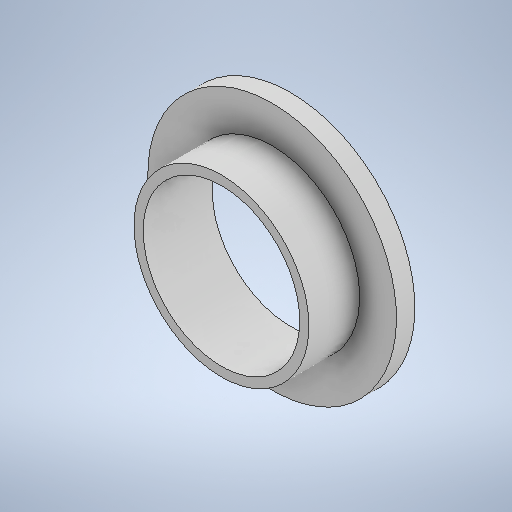
# Autodesk Inventor part: Ø10-Ø8Prop
Saved by Autodesk Inventor 2025.1 (Build 291241000, 241)
## iProperties
Created: 2025-02-27
Part Number: Ø10-Ø8Prop
Material: Generic
Document SubType Name: Modeling
Designer: frede
Density: 1 g/cm^3
Appearance: Default
Author: frede
Autodesk Inventor part; units mm, degrees
ref_plane "YZ Plane" through (0, 0, 0) normal (1, 0, 0) x (0, 1, 0)
ref_plane "XZ Plane" through (0, 0, 0) normal (0, 1, 0) x (-1, 0, 0)
ref_plane "XY Plane" through (0, 0, 0) normal (0, 0, 1) x (1, 0, 0)
sketch "Sketch1" plane through (0, 0, 0) normal (1, 0, 0) x (0, 1, 0)
  line L0 (4.25, 0) -> (4.25, -3.75)
  line L1 (0, -2.75) -> (0, 0)
  line L2 (4.75, -2.75) -> (4.75, 0)
  line L3 (4.75, 0) -> (4.25, 0)
  line L4 (4.25, 0) -> (4.25, -2.75)
  line L5 (6.75, -2.75) -> (6.75, -3.75)
  line L6 (6.75, -3.75) -> (4.25, -3.75)
  line L7 (4.75, -2.75) -> (6.75, -2.75)
  point P0 (4.1, 0)
  dimension "d3" = 2.5
  dimension "d4" = 1
  dimension "d5" = 2.75
  dimension "d6" = 4.75
  dimension "d8" = 4.25
  constraints: 16 end point, 2 parallel, 1 horizontal, 1 point on line
  measures "d3" distance of L0.end L5.end
  measures "d4" distance of L5.start L5.end
  measures "d5" distance between parallel lines of L7 L3
  measures "d6" distance between parallel lines of L1 L2
  measures "d8" distance between parallel lines of L1 L0
revolve "Revolution1" add sketch "Sketch1" angle 360 about axis through (0, 0, -2.75) along (0, 0, 1)
body "Solid1"
